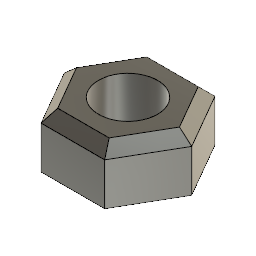
M6_Pneumatic_Nut (Autodesk Fusion 360 design; units mm, degrees)
Autodesk Fusion 360 part; units mm, degrees
sketch "Sketch1" plane through (0, 0, 0) normal (0, 0, 1) x (1, 0, 0) in component "Pneumatic Nut"
  line L0 (-3, 5.1962) -> (-6, 0)
  line L1 (-6, 0) -> (-3, -5.1962)
  line L2 (-3, -5.1962) -> (3, -5.1962)
  line L3 (3, -5.1962) -> (6, 0)
  line L4 (6, 0) -> (3, 5.1962)
  line L5 (3, 5.1962) -> (-3, 5.1962)
  circle A0 centre (0, 0) radius 2.775
  dimension "d1" = 12
  dimension "d2" = 5.55
  measures "d2" diameter of A0
extrude "Extrude1" add sketch "Sketch1" along normal blind 5 in component "Pneumatic Nut"
chamfer "Chamfer1" distance 1 angle 45 6 edges at (4.5, -2.5981, 5) (4.5, 2.5981, 5) (0, 5.1962, 5) (-4.5, 2.5981, 5) (-4.5, -2.5981, 5) (0, -5.1962, 5) in component "Pneumatic Nut"
component "Pneumatic Nut" placed x (1, 0, 0) y (0, 1, 0) z (0, 0, 1) at (0, 0, 0)
